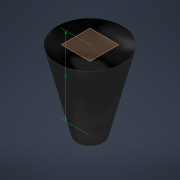
# Autodesk Inventor part: Soportes
Saved by Autodesk Inventor 2021 (Build 250183000, 183)
## iProperties
Created: 2021-03-29
Part Number: Soportes
Material: Genérico
Document SubType Name: Modeling
Designer: grego
Density: 1 g/cm^3
Appearance: Valor por defecto
Author: grego
Autodesk Inventor part; units mm, degrees
ref_plane "YZ Plane" through (0, 0, 0) normal (1, 0, 0) x (0, 1, 0)
ref_plane "XY Plane" through (0, 0, 0) normal (0, 0, 1) x (1, 0, 0)
sketch "Boceto1" plane through (0, 0, 0) normal (0, 1, 0) x (-1, 0, 0)
  circle A0 centre (0, 0) radius 1
  dimension "d0" = 2
  constraints: 1 centre point, 1 coincident
  measures "d0" diameter of A0
sketch "Boceto2" plane through (0, 0, 0) normal (0, 0, 1) x (1, 0, 0)
  line L0 (0, 0) -> (0, 6)
  dimension "d1" = 6
  constraints: 2 end point, 1 vertical
  measures "d1" distance of L0.start L0.end
ref_plane "Plano de trabajo1" through (0, 6, 0) normal (0, 1, 0) x (-1, 0, 0)
sketch "Boceto3" plane through (0, 6, 0) normal (0, 1, 0) x (-1, 0, 0)
  circle A0 centre (0, 0) radius 2.5
  dimension "d3" = 5
  constraints: 1 centre point, 1 coincident
  measures "d3" diameter of A0
loft "Solevación1" add profiles "Boceto3", "Boceto1"
